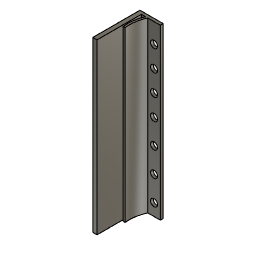
screwdriver holder v1 (Autodesk Fusion 360 design; units mm, degrees)
Autodesk Fusion 360 part; units mm, degrees
sketch "Sketch1" plane through (0, 0, 0) normal (0, 0, 1) x (1, 0, 0) in component "Component"
  line L0 (0, 0) -> (6, 0)
  line L1 (6, 0) -> (6, -67)
  line L2 (6, -67) -> (0, -67)
  line L3 (0, -67) -> (0, 0)
  line L4 (6, 0) -> (18, 0)
  line L5 (18, 0) -> (18, -4)
  line L6 (18, -4) -> (6, -4)
  line L7 (6, -4) -> (6, 0)
  line L8 (8.0693, -4) -> (8.0693, -32) construction
  arc A0 (12, -4) -> (8.0693, -32) centre (59.8982, -25) ccw
  arc A1 (15.1021, -4) -> (10.8522, -32) centre (61.2859, -25.3325) ccw
  line L9 (8.0693, -32) -> (10.8522, -32)
  dimension "d1" = 6
  dimension "d2" = 67
  dimension "d3" = 12
  dimension "d4" = 4
  dimension "d5" = 28
  constraint horizontal L0
  constraint vertical L1
  constraint horizontal L2
  constraint vertical L3
  constraint coincident L0.start L3.end
  constraint horizontal L4
  constraint vertical L5
  constraint horizontal L6
  constraint vertical L7
  constraint coincident L6 L8.start
  constraint perpendicular L6 L8
  constraint midpoint L6 A0.start
  constraint tangent A0 A1
  constraint coincident L6 A1.start
  constraint perpendicular L8 L9
  measures "d1" distance of L0.start L0.end
  measures "d2" distance of L0.start L2.end
  measures "d3" distance of L0.end L4.end
  measures "d4" distance of L0.end L6.end
  measures "d5" distance of L8.start L8.end
extrude "Extrude1" add sketch "Sketch1" along normal blind 240 in component "Component"
sketch "Sketch2" plane through (0, 0, 0) normal (0, 1, 0) x (-1, 0, 0) in component "Component"
  line L0 (-18, 0) -> (0, 0)
  line L1 (0, 0) -> (0, 240)
  line L2 (0, 240) -> (-18, 240)
  line L3 (-18, 240) -> (-18, 0)
  circle A0 centre (-24, 17) radius 5
  line L4 (-9, 47) -> (-24, 52) construction
  circle A1 centre (-24, 52) radius 5
  circle A2 centre (-24, 87) radius 5
  circle A3 centre (-24, 122) radius 5
  circle A4 centre (-24, 152) radius 5
  circle A5 centre (-24, 182) radius 5
  circle A6 centre (-24, 212) radius 5
  dimension "d10" = 10
  dimension "d12" = 10
  dimension "d14" = 10
  dimension "d16" = 10
  dimension "d18" = 10
  dimension "d20" = 10
  dimension "d22" = 10
  constraint coincident L4.end A1.centre
  measures "d10" diameter of A0
  measures "d12" diameter of A1
  measures "d14" diameter of A2
  measures "d16" diameter of A3
  measures "d18" diameter of A4
  measures "d20" diameter of A5
  measures "d22" diameter of A6
sketch "Sketch3" plane through (0, 0, 0) normal (0, 0, 1) x (1, 0, 0) in component "Component"
  line L0 (18, 0) -> (33, 0)
  line L1 (18, -4) -> (33, -4)
  line L2 (33, -4) -> (33, 0)
  line L3 (18, 0) -> (18, -4)
  dimension "d23" = 15
  constraint horizontal L0
  constraint horizontal L1
  constraint perpendicular L1 L3
  measures "d23" distance of L0.start L0.end
extrude "Extrude2" add sketch "Sketch3" along normal blind 240 in component "Component"
extrude "Extrude3" cut sketch "Sketch2" against normal blind 20 contours A0 | A1 | A2 | A3 | A4 | A5 | A6 in component "Component"
component "Component" placed x (1, 0, 0) y (0, 1, 0) z (0, 0, 1) at (0, 0, 0)
